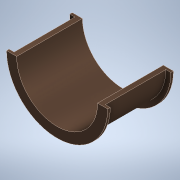
# Autodesk Inventor part: Верхняя часть коренного подшипника
Saved by Autodesk Inventor 2021 (Build 250183000, 183)
## iProperties
Created: 2020-12-05
Part Number: Верхняя часть коренного подшипника
Material: Бронза, литейная
Document SubType Name: Modeling
Designer: Тимоха
Mass: 2835.31 g
Surface Area: 719.857 cm^2
Volume: 319.652 cm^3
Density: 8.87 g/cm^3
Appearance: Бронза - сатинированная
Author: Тимоха
Autodesk Inventor part; units mm, degrees
ref_plane "YZ Plane" through (0, 0, 0) normal (1, 0, 0) x (0, 1, 0)
ref_plane "XZ Plane" through (0, 0, 0) normal (0, 1, 0) x (-1, 0, 0)
sketch "Эскиз1" plane through (0, 0, 0) normal (0, 0, 1) x (1, 0, 0)
  circle A0 centre (0, 0) radius 80
  circle A1 centre (0, 0) radius 90
  line L0 (-90, 0) -> (90, 0)
  point P0 (-80, 0)
  point P1 (80, 0)
  dimension "d0" = 160
  dimension "d1" = 180
  constraints: 2 centre point, 2 coincident, 2 end point, 2 point on circle, 1 horizontal
  measures "d0" diameter of A0
  measures "d1" diameter of A1
extrude "Выдавливание1" add sketch "Эскиз1" along normal blind 120 contours L0 A1 A0 picked at (54.1763, -63.1025)
sketch "Эскиз3" plane through (0, 0, 120) normal (0, 0, 1) x (1, 0, 0)
  arc A0 (-90, 0) -> (90, 0) centre (0, 0) ccw projected
  line L0 (90, 0) -> (80, 0) projected
  arc A1 (-80, 0) -> (80, 0) centre (0, 0) ccw projected
  line L1 (-80, 0) -> (-90, 0) projected
  circle A2 centre (0, 0) radius 100
  arc A3 (-90, 0) -> (90, 0) centre (0, 0) ccw projected
  line L2 (-90, 0) -> (-100, 0)
  line L3 (90, 0) -> (100, 0)
  dimension "d7" = 200
  constraints: 4 end point, 2 point on circle, 1 centre point, 1 coincident, 1 point on line
  measures "d7" diameter of A2
extrude "Выдавливание3" add sketch "Эскиз3" along normal blind 5 contours L1 A1 L0 A0 | A0 L3 A2 L2
ref_plane "РабПлоскость2" through (0, 0, 60) normal (0, 0, -1) x (-1, 0, 0)
mirror "Зеркальное отражение1" about plane through (0, 0, 60) normal (0, 0, -1) of "Выдавливание3"
